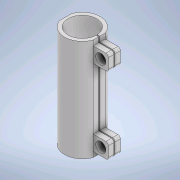
# Autodesk Inventor part: Hülse
Saved by Autodesk Inventor 2020.1 (Build 241239000, 239)
## iProperties
Created: 2020-08-17
Part Number: Hülse
Material: Generisch
Document SubType Name: Modeling
Designer: s5chfeis
Density: 1 g/cm^3
Appearance: Vorgabe
Author: s5chfeis
Autodesk Inventor part; units mm, degrees
ref_plane "YZ Plane" through (0, 0, 0) normal (1, 0, 0) x (0, 1, 0)
ref_plane "XZ Plane" through (0, 0, 0) normal (0, 1, 0) x (-1, 0, 0)
ref_plane "XY Plane" through (0, 0, 0) normal (0, 0, 1) x (1, 0, 0)
sketch "Skizze1" plane through (0, 0, 0) normal (0, 1, 0) x (-1, 0, 0)
  circle A0 centre (0, 0) radius 14
  circle A1 centre (0, 0) radius 17.5
  dimension "d0" = 28
  dimension "d1" = 35
  constraints: 2 centre point, 2 coincident
  measures "d0" diameter of A0
  measures "d1" diameter of A1
extrude "Extrusion1" add sketch "Skizze1" along normal blind 100
sketch "Skizze2" plane through (0, 100, 0) normal (0, 1, 0) x (1, 0, 0)
  circle A0 centre (0, 0) radius 17.5 construction
  line L0 (-17.5, 0) -> (17.5, 0) construction
  line L1 (0, -17.5) -> (0, 17.5) construction
  line L2 (11.1238, 0) -> (19.1238, 0)
  line L3 (19.1238, 0) -> (19.1238, 0.5)
  line L4 (19.1238, 0.5) -> (11.1238, 0.5)
  line L5 (11.1238, 0.5) -> (11.1238, 0)
  line L6 (11.1238, 0) -> (19.1238, 0)
  line L7 (19.1238, 0) -> (19.1238, -0.5)
  line L8 (19.1238, -0.5) -> (11.1238, -0.5)
  line L9 (11.1238, -0.5) -> (11.1238, 0)
  dimension "d4" = 8
  dimension "d5" = 0.5
  dimension "d6" = 0.5
  constraints: 20 end point, 4 parallel, 4 point on circle, 3 horizontal, 2 perpendicular, 2 point on line
  measures "d4" distance of L4.end L3.end
  measures "d5" distance of L3.end L2.end
  measures "d6" distance of L6.end L7.end
extrude "Extrusion2" cut sketch "Skizze2" against normal blind 1000
sketch "Skizze3" plane through (0, 100, 0) normal (0, 1, 0) x (1, 0, 0)
  arc A0 (17.4929, 0.5) -> (17.4929, -0.5) centre (0, 0) ccw construction
  line L0 (-17.5, 0) -> (17.4929, 0) construction
  line L1 (-17.5, 0) -> (-16.5, 0)
  line L2 (-16.5, 0) -> (-16.5, 10)
  line L3 (-16.5, 10) -> (-17.5, 10)
  line L4 (-17.5, 10) -> (-17.5, 0)
  line L5 (-17.5, 0) -> (-16.5, 0)
  line L6 (-16.5, 0) -> (-16.5, -14.1837)
  line L7 (-16.5, -14.1837) -> (-17.5, -14.1837)
  line L8 (-17.5, -14.1837) -> (-17.5, 0)
  line L9 (-0.0036, -17.5) -> (-0.0036, 17.5) construction
  line L10 (17.4929, 0) -> (16.4929, 0)
  line L11 (16.4929, 0) -> (16.4929, 10)
  line L12 (16.4929, 10) -> (17.4929, 10)
  line L13 (17.4929, 10) -> (17.4929, 0)
  line L14 (17.4929, 0) -> (16.4929, 0)
  line L15 (16.4929, 0) -> (16.4929, -14.1837)
  line L16 (16.4929, -14.1837) -> (17.4929, -14.1837)
  line L17 (17.4929, -14.1837) -> (17.4929, 0)
  dimension "d9" = 1
  dimension "d10" = 10
  constraints: 36 end point, 6 symmetric about line, 4 parallel, 3 horizontal, 3 point on circle, 2 perpendicular, 2 point on line, 1 vertical
  measures "d9" distance of L3.end L2.end
  measures "d10" distance of L2.end L1.end
extrude "Extrusion3" cut sketch "Skizze3" against normal blind 1000
sketch "Skizze4" plane through (16.4929, 100, 5.8511) normal (1, 0, 0) x (0, 0, -1)
  line L0 (0, -100) -> (0, 0) projected
  line L1 (5.3511, 0) -> (0, 0)
  line L2 (0, 0) -> (0, -5)
  line L3 (0, -5) -> (5.3511, -5)
  line L4 (5.3511, -5) -> (5.3511, 0)
  line L5 (0, -5) -> (5.3511, -5)
  line L6 (5.3511, -5) -> (5.3511, -20)
  line L7 (5.3511, -20) -> (0, -20)
  line L8 (0, -20) -> (0, -5)
  line L9 (11.7023, 0) -> (11.7023, -100) projected
  line L10 (6.3511, 0) -> (11.7023, 0)
  line L11 (11.7023, 0) -> (11.7023, -5)
  line L12 (11.7023, -5) -> (6.3511, -5)
  line L13 (6.3511, -5) -> (6.3511, 0)
  line L14 (6.3511, -5) -> (11.7023, -5)
  line L15 (11.7023, -5) -> (11.7023, -20)
  line L16 (11.7023, -20) -> (6.3511, -20)
  line L17 (6.3511, -20) -> (6.3511, -5)
  line L18 (0, -50) -> (11.7023, -50) construction
  line L19 (5.3511, -100) -> (0, -100)
  line L20 (0, -100) -> (0, -95)
  line L21 (0, -95) -> (5.3511, -95)
  line L22 (5.3511, -95) -> (5.3511, -100)
  line L23 (0, -95) -> (5.3511, -95)
  line L24 (5.3511, -95) -> (5.3511, -80)
  line L25 (5.3511, -80) -> (0, -80)
  line L26 (0, -80) -> (0, -95)
  line L27 (6.3511, -100) -> (11.7023, -100)
  line L28 (11.7023, -100) -> (11.7023, -95)
  line L29 (11.7023, -95) -> (6.3511, -95)
  line L30 (6.3511, -95) -> (6.3511, -100)
  line L31 (6.3511, -95) -> (11.7023, -95)
  line L32 (11.7023, -95) -> (11.7023, -80)
  line L33 (11.7023, -80) -> (6.3511, -80)
  line L34 (6.3511, -80) -> (6.3511, -95)
  point P0 (5.8511, -100)
  point P1 (11.7023, -80)
  point P2 (0, -80)
  dimension "d13" = 5
  dimension "d14" = 15
  dimension "d15" = 15
  constraints: 66 end point, 16 symmetric about line, 8 parallel, 7 point on line, 4 horizontal, 4 perpendicular, 2 midpoint
  measures "d13" distance of L2.end L1.end
  measures "d14" distance of L5.end L6.end
  measures "d15" distance of L14.end L15.end
extrude "Extrusion4" add sketch "Skizze4" along normal blind 15 contours L0 L3 L6 L7 | L0 L25 L24 L21 | L9 L29 L34 L33 | L9 L16 L17 L12
fillet "Rundung1" radius 2.5 8 edges at (31.4929, 95, 3.1756) (31.4929, 80, 3.1756) (31.4929, 80, -3.1756) (31.4929, 95, -3.1756) (31.4929, 20, 3.1756) (31.4929, 5, 3.1756) (31.4929, 20, -3.1756) (31.4929, 5, -3.1756)
sketch "Skizze5" plane through (16.4929, 80, 5.8511) normal (0, 0, 1) x (1, 0, 0)
  line L0 (0, 0) -> (12.5, 0) construction
  line L1 (0, 0) -> (7.5, 0) construction
  line L2 (0, 0) -> (7.5, 0) construction
  line L3 (7.5, 0) -> (7.5, 7.5) construction
  circle A0 centre (7.5, 7.5) radius 5
  line L4 (0, -75) -> (12.5, -75) construction
  line L5 (0, -75) -> (7.5, -75) construction
  line L6 (0, -75) -> (7.5, -75) construction
  line L7 (7.5, -75) -> (7.5, -67.5) construction
  circle A1 centre (7.5, -67.5) radius 5
  point P0 (-16.4929, -80)
  dimension "d19" = 7.5
  dimension "d20" = 0
  dimension "d21" = 7.5
  dimension "d22" = 90
  dimension "d23" = 10
  dimension "d24" = 7.5
  dimension "d25" = 0
  dimension "d26" = 7.5
  dimension "d27" = 90
  dimension "d28" = 10
  constraints: 12 end point, 4 collinear, 2 centre point, 2 coincident, 2 horizontal, 2 perpendicular
  measures "d19" distance of L0.start L1.end
  measures "d20" distance between parallel lines of L1 L2
  measures "d21" distance of L1.end L3.end
  measures "d22" angle of L3 L1
  measures "d23" diameter of A0
  measures "d24" distance of L4.start L5.end
  measures "d25" distance between parallel lines of L5 L6
  measures "d26" distance of L5.end L7.end
  measures "d27" angle of L7 L5
  measures "d28" diameter of A1
extrude "Extrusion5" cut sketch "Skizze5" against normal blind 100
